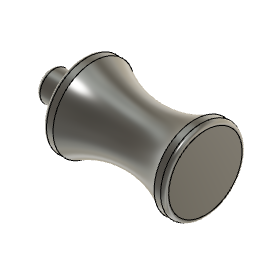
pion_toile_amorce (Autodesk Fusion 360 design; units mm, degrees)
Autodesk Fusion 360 part; units mm, degrees
sketch "Esquisse1" plane through (0, 0, 0) normal (0, 0, 1) x (1, 0, 0)
  line L0 (0, 0) -> (25, 0) construction
  line L1 (0, 0) -> (0, 1.8)
  line L2 (0, 1.8) -> (4, 1.8)
  line L3 (4, 1.8) -> (4, 5)
  line L4 (4, 5) -> (19, 5)
  line L5 (19, 5) -> (19, 0)
  arc A0 (5.3, 5) -> (17.7, 5) centre (11.5, 15.4559) ccw
  line L6 (0, 0) -> (19, 0)
  line L7 (7.6902, 3.3) -> (16, 3.3) construction
  dimension "d1" = 1.8
  dimension "d2" = 4
  dimension "d3" = 5
  dimension "d4" = 1.3
  dimension "d5" = 1.3
  dimension "d12" = 15
  dimension "d14" = 3.3
  constraint coincident L0.start L1.start
  constraint horizontal L0
  constraint vertical L1
  constraint perpendicular L1 L2
  constraint perpendicular L2 L3
  constraint perpendicular L3 L4
  constraint coincident L0 L5.end
  constraint perpendicular L0 L5
  constraint coincident L4 A0.end
  constraint coincident L4 A0.start
  constraint tangent A0 L7
  constraint parallel L6 L7
  measures "d1" distance of L0.start L1.end
  measures "d2" distance of L1.end L2.end
  measures "d3" distance of L0 L4
  measures "d4" distance of L3.end A0.start
  measures "d5" distance of L4.end A0.end
  measures "d12" distance of L3 L5
  measures "d14" distance of L6 L7
revolve "Révolution1" add sketch "Esquisse1" angle 360 about axis through (0, 0, 0) along (1, 0, 0) contours L1 L2 L3 L4 L5 A0 L6
fillet "Congé1" radius 0.5 2 edges at (19, -1.8081, 4.6616) (4, -1.8081, 4.6616)
fillet "Congé2" radius 0.5 1 edges at (0, -0.6509, 1.6782)
